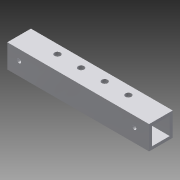
# Autodesk Inventor part: 1x1 pickup arm support rear
Saved by Autodesk Inventor 2015 SP1 (Build 190203100, 203)
## iProperties
Created: 2015-01-27
Part Number: 1x1 pickup arm support rear
Material: Aluminum 6061
Document SubType Name: Modeling
Designer: Admin
Density: 2.7 g/cm^3
Appearance: Aluminum - Flat
Author: Admin
Autodesk Inventor part; units mm, degrees
ref_plane "YZ Plane" through (0, 0, 0) normal (1, 0, 0) x (0, 1, 0)
ref_plane "XZ Plane" through (0, 0, 0) normal (0, 1, 0) x (-1, 0, 0)
ref_plane "XY Plane" through (0, 0, 0) normal (0, 0, 1) x (1, 0, 0)
sketch "Sketch1" plane through (0, 0, 0) normal (1, 0, 0) x (0, 1, 0)
  line L0 (0, 0) -> (25.4, 0)
  line L1 (25.4, 0) -> (25.4, -25.4)
  line L2 (25.4, -25.4) -> (0, -25.4)
  line L3 (0, -25.4) -> (0, 0)
  line L4 (3.175, -3.175) -> (22.225, -3.175)
  line L5 (22.225, -3.175) -> (22.225, -22.225)
  line L6 (22.225, -22.225) -> (3.175, -22.225)
  line L7 (3.175, -22.225) -> (3.175, -3.175)
  dimension "d0" = 25.4
  dimension "d1" = 25.4
  dimension "d2" = 19.05
  dimension "d3" = 19.05
  dimension "d4" = 3.175
  dimension "d5" = 3.175
  constraints: 16 end point, 4 parallel, 2 horizontal, 2 perpendicular
  measures "d0" distance of L1.end L2.end
  measures "d1" distance of L0.end L1.end
  measures "d2" distance of L5.end L6.end
  measures "d3" distance of L4.end L5.end
  measures "d4" distance between parallel lines of L3 L7
  measures "d5" distance between parallel lines of L0 L4
extrude "Extrusion1" add sketch "Sketch1" along normal blind 152.4
sketch "Sketch2" plane through (0, 25.4, 0) normal (0, 1, 0) x (1, 0, 0)
  line L0 (0, 0) -> (0, 25.4) projected
  line L1 (0, 0) -> (152.4, 0) projected
  line L2 (152.4, 25.4) -> (152.4, 0) projected
  point P0 (38.1, 15.875)
  point P1 (114.3, 15.875)
  dimension "d8" = 38.1
  dimension "d9" = 15.875
  dimension "d10" = 15.875
  dimension "d11" = 38.1
  measures "d8" distance from line of point (38.1, 15.875) L0
  measures "d9" distance from line of L1 point (38.1, 15.875)
  measures "d10" distance from line of L1 point (114.3, 15.875)
  measures "d11" distance from line of L2 point (114.3, 15.875)
hole "Hole1" at (38.1, 25.4, -15.875) at (114.3, 25.4, -15.875) direction (0, -1, 0) diameter 6.35 end through all
sketch "Sketch3" plane through (0, 0, 0) normal (0, 0, 1) x (1, 0, 0)
  line L0 (0, 0) -> (0, 25.4) projected
  line L1 (0, 0) -> (152.4, 0) projected
  line L2 (152.4, 25.4) -> (152.4, 0) projected
  point P0 (12.7, 14.2875)
  point P1 (136.525, 14.2875)
  dimension "d19" = 15.875
  dimension "d20" = 14.2875
  dimension "d21" = 12.7
  dimension "d22" = 14.2875
  measures "d19" distance from line of L2 point (136.525, 14.287)
  measures "d20" distance from line of L1 point (136.525, 14.287)
  measures "d21" distance from line of L0 point (12.7, 14.287)
  measures "d22" distance from line of L1 point (12.7, 14.287)
hole "Hole2" at (12.7, 14.2875, 0) at (136.525, 14.2875, 0) direction (0, 0, -1) diameter 4.3656 end through all
sketch "Sketch4" plane through (0, 25.4, 0) normal (0, 1, 0) x (1, 0, 0)
  line L0 (0, 0) -> (152.4, 0) projected
  line L1 (0, 0) -> (0, 25.4) projected
  point P0 (63.5, 15.875)
  dimension "d30" = 15.875
  dimension "d39" = 63.5
  measures "d30" distance from line of L0 point (63.5, 15.875)
  measures "d39" distance from line of point (63.5, 15.875) L1
hole "Hole3" at (63.5, 25.4, -15.875) direction (0, -1, 0) diameter 6.35 end through all
sketch "Sketch5" plane through (0, 25.4, 0) normal (0, 1, 0) x (1, 0, 0)
  circle A0 centre (114.3, 15.875) radius 3.175 projected
  line L0 (0, 25.4) -> (152.4, 25.4) projected
  point P0 (88.9, 15.875)
  dimension "d40" = 9.525
  dimension "d41" = 25.4
  measures "d40" distance from line of L0 point (88.9, 15.875)
  measures "d41" distance of A0.centre point (88.9, 15.875)
hole "Hole4" at (88.9, 25.4, -15.875) direction (0, -1, 0) diameter 6.35 depth 25.4 tip angle 118
body "Solid1"
